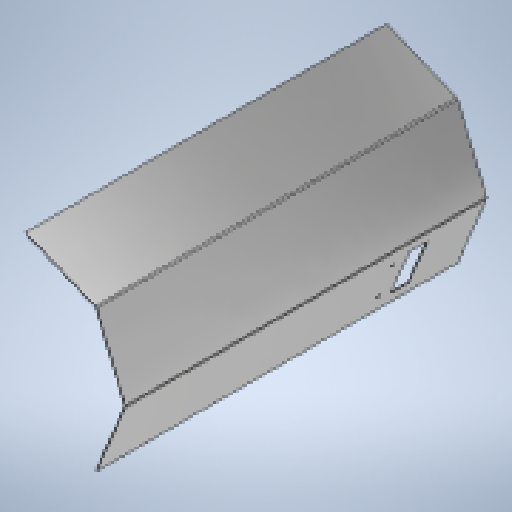
# Autodesk Inventor part: DMF 01 14 Барабан Лист прав брт v2.1
Saved by Autodesk Inventor 2025.3 (Build 293356000, 356)
## iProperties
Created: 2024-04-28
Part Number: DMF 01 14 Барабан Лист прав брт v2.1
Material: Stainless Steel AISI 304
Document SubType Name: Sheet Metal
Designer: pokla
Density: 8 g/cm^3
Appearance: Chrome - Satin
Sheet Metal Rule: Default
Flat Pattern Width: 63.5199 cm
Flat Pattern Length: 100 cm
Flat Pattern Area: 6351.99 cm^2
Sheet Metal Width: 635,199 mm
Sheet Metal Length: 1000,000 mm
Sheet Metal Area: 635199,033 mm^2
Stock Number: Барабан_Лист_Правый_Борт
Author: pokla
Autodesk Inventor part; units mm, degrees
ref_plane "YZ Plane" through (0, 0, 0) normal (1, 0, 0) x (0, 1, 0)
ref_plane "XZ Plane" through (0, 0, 0) normal (0, 1, 0) x (-1, 0, 0)
ref_plane "XY Plane" through (0, 0, 0) normal (0, 0, 1) x (1, 0, 0)
sketch "Sketch2" plane through (0, 0, 0) normal (0, 0, 1) x (1, 0, 0)
  line L0 (0, 277.633599) -> (196.316601, 196.316601) construction
  line L1 (196.316601, 196.316601) -> (277.633599, 0) construction
  line L2 (277.633599, 0) -> (196.316601, -196.316601) construction
  line L3 (196.316601, -196.316601) -> (0, -277.633599) construction
  line L4 (0, -277.633599) -> (-196.316601, -196.316601) construction
  line L5 (-196.316601, -196.316601) -> (-277.633599, 0) construction
  line L6 (-277.633599, 0) -> (-196.316601, 196.316601) construction
  line L7 (-196.316601, 196.316601) -> (0, 277.633599) construction
  line L8 (196.950651, 194.785867) -> (276.999549, 1.530734)
  line L9 (276.999549, -1.530734) -> (196.950651, -194.785867)
  arc A0 (276.999549, -1.530734) -> (276.999549, 1.530734) centre (273.304031, 0) ccw
  line L10 (194.785867, -196.950651) -> (0.831492, -277.289184) construction
  arc A1 (194.785867, -196.950651) -> (196.950651, -194.785867) centre (193.255133, -193.255133) ccw construction
  line L11 (277.633599, 0) -> (276.999549, 1.530734) construction
  line L12 (276.999549, 1.530734) -> (278.530282, 2.164784) construction
  line L13 (278.530282, 2.164784) -> (279.164333, 0.634051) construction
  line L14 (279.164333, 0.634051) -> (277.633599, 0) construction
  line L15 (194.785867, 196.950651) -> (1.530734, 276.999549)
  arc A2 (196.950651, 194.785867) -> (194.785867, 196.950651) centre (193.255133, 193.255133) ccw
  line L16 (1.530734, 276.999549) -> (0, 277.633599) construction
  line L17 (0, 277.633599) -> (0.634051, 279.164333) construction
  line L18 (0.634051, 279.164333) -> (2.164784, 278.530282) construction
  line L19 (2.164784, 278.530282) -> (1.530734, 276.999549) construction
  point P0 (0, 0)
  point P1 (0, 0)
  dimension "d56" = 513
  dimension "d58" = 4
  dimension "d69" = 0.9
  dimension "d70" = 4
  measures "d56" distance between parallel lines of L6 L2
  measures "d58" radius of A0
  measures "d69" distance of L3.end L10.end
  measures "d70" radius of A1
contour flange "Contour Flange2" sketch "Sketch2" thickness 2 bend radius 2 width 1000 along (0, 0, 1) mid plane no both sides no wall seen from (98.1583, 236.9751, 0) lies toward (0.3826834, 0.9238795, 0) curves L15 A2 L8 A0 L9
bend "Bend2"
corner "Corner2"
sketch "Sketch11" plane through (278.847308, 2.296101, 1000) normal (0.9238795, 0.3826834, 0) x (0, 0, -1)
  line L0 (900, 154.588924) -> (950, 154.588924)
  line L1 (950, 154.588924) -> (950, 54.588924)
  line L2 (950, 54.588924) -> (900, 54.588924)
  line L3 (900, 54.588924) -> (900, 154.588924)
  circle A0 centre (880, 154.588924) radius 4.5
  circle A1 centre (880, 54.588924) radius 4.5
  line L4 (950, 104.588924) -> (900, 104.588924) construction
  line L5 (1000, 209.177849) -> (1000, 0)
  point P0 (1000, 104.588924)
  point P1 (1000, 104.588924)
  dimension "d132" = 9
  dimension "d133" = 100
  dimension "d134" = 50
  dimension "d135" = 20
  dimension "d136" = 50
  dimension "d137" = 100
  constraints: 10 end point, 3 midpoint, 2 centre point, 2 parallel, 1 horizontal, 1 perpendicular, 1 point on line, 1 other
  measures "d132" diameter of A0
  measures "d133" distance of L2.end L0.start
  measures "d134" distance of L0.start L0.end
  measures "d135" distance from line of A0.centre L3
  measures "d136" distance between parallel lines of L5 L1
  measures "d137" distance of A1.centre A0.centre
extrude "Cut1" cut sketch "Sketch11" against normal blind 2
equation "\"d56\" = Барабан_габарит_по_кассетам"
equation "\"d58\" = BendRadius + Thickness"
equation "\"d69\" = Барабан_отступ_развертки"
equation "\"d70\" = BendRadius + Thickness"
equation "\"d25\" = Thickness"
equation "\"d26\" = BendReliefWidth"
equation "\"d27\" = BendReliefDepth"
equation "\"d28\" = MinimumRemnant"
equation "\"d29\" = TransitionRadius"
equation "\"d31\" = BendRadius"
equation "\"d33\" = CornerReliefSize"
equation "\"d34\" = GapSize"
equation "\"d35\" = JacobiRadiusSize"
equation "\"BendRadius\" = Thickness"
equation "\"BendReliefWidth\" = Thickness"
equation "\"BendReliefDepth\" = 0.5 * Thickness"
equation "\"CornerReliefSize\" = 4 * Thickness"
equation "\"MinimumRemnant\" = 2 * Thickness"
equation "\"TransitionRadius\" = BendRadius"
equation "\"JacobiRadiusSize\" = BendRadius"
equation "\"GapSize\" = Thickness"
equation "\"Барабан_габарит_по_кассетам\" = 513"
equation "\"Thickness\" = 2"
equation "\"Барабан_отступ_развертки\" = 0.9"
body "Solid2"
